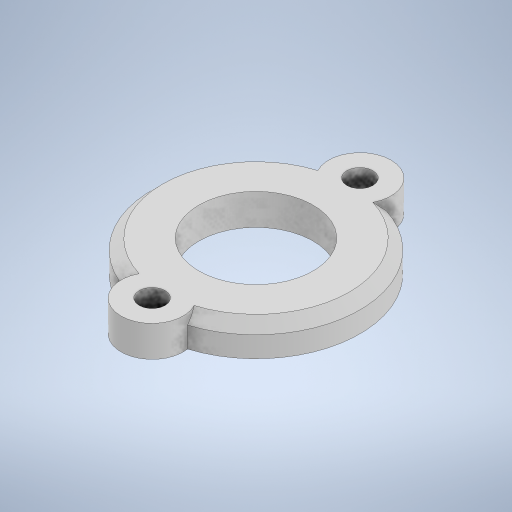
# Autodesk Inventor part: 책상 고정판 홀더
Saved by Autodesk Inventor 2023 (Build 270158000, 158)
## iProperties
Created: 2022-11-11
Part Number: 책상 고정판 홀더
Material: 일반
Document SubType Name: Modeling
Designer: hyunsu
Density: 1 g/cm^3
Appearance: 기본값
Author: hyunsu
Autodesk Inventor part; units mm, degrees
ref_plane "YZ Plane" through (0, 0, 0) normal (1, 0, 0) x (0, 1, 0)
ref_plane "XZ Plane" through (0, 0, 0) normal (0, 1, 0) x (-1, 0, 0)
ref_plane "XY Plane" through (0, 0, 0) normal (0, 0, 1) x (1, 0, 0)
sketch "스케치1" plane through (0, 0, 0) normal (0, 1, 0) x (-1, 0, 0)
  circle A0 centre (0, 0) radius 10
  circle A1 centre (0, 10) radius 1.25
  circle A2 centre (0, 10) radius 3
  line L0 (0, 0) -> (3.5124, 0)
  circle A3 centre (0, -10) radius 1.25
  circle A4 centre (0, -10) radius 3
  circle A5 centre (0, 0) radius 5.5
  point P0 (2.9661, 9.55)
  point P1 (-2.9661, 9.55)
  point P2 (-2.9661, -9.55)
  point P3 (2.9661, -9.55)
  dimension "d0" = 20
  dimension "d2" = 2.5
  dimension "d3" = 6
  dimension "d4" = 11
  constraints: 5 centre point, 4 coincident, 2 end point, 2 symmetric about line, 1 horizontal, 1 vertical alignment, 5 other
  measures "d2" diameter of A1
  measures "d3" diameter of A2
  measures "d4" diameter of A5
extrude "돌출1" add sketch "스케치1" along normal blind 3 contours A0 A4 A2 | A2 A0 A1 | A0 A1 A2 | A4 A0 A3 | A0 A3 A4
chamfer "모따기1" distance 1 angle 45 2 edges at (10, 3, 0) (-10, 3, 0)
